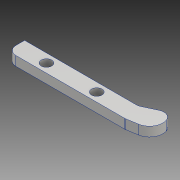
# Autodesk Inventor part: phalanx_1_tendon_support
Saved by Autodesk Inventor 2017 SP1 (Build 210196100, 196)
## iProperties
Created: 2017-07-31
Part Number: phalanx_1_tendon_support
Material: Aluminum 6061
Document SubType Name: Modeling
Designer: JT
Density: 2.7 g/cm^3
Appearance: Aluminum - Flat
Author: JT
Autodesk Inventor part; units mm, degrees
ref_plane "YZ Plane" through (0, 0, 0) normal (1, 0, 0) x (0, 1, 0)
ref_plane "XZ Plane" through (0, 0, 0) normal (0, 1, 0) x (-1, 0, 0)
ref_plane "XY Plane" through (0, 0, 0) normal (0, 0, 1) x (1, 0, 0)
sketch "Sketch1" plane through (0, 0, 0) normal (0, 0, 1) x (1, 0, 0)
  line L0 (0, 4) -> (0, 0) construction
  arc A0 (8.3449, 0.4035) -> (9.5, 6.1037) centre (8.2, 3.4) ccw
  line L1 (0, 0) -> (-21, 0)
  line L2 (-21, 0) -> (-21, 4)
  line L3 (0, 4) -> (0, 0)
  line L4 (-21, 4) -> (0, 4)
  line L5 (0, 4) -> (5, 4)
  line L6 (5, 4) -> (9.5, 6.1037)
  line L7 (0, 0) -> (6, 0)
  line L8 (6, 0) -> (8.6846, 0.4394)
  dimension "d0" = 8.2
  dimension "d1" = 3.4
  dimension "d3" = 6
  dimension "d47" = 21
  dimension "d57" = 4
  dimension "d66" = 5
  dimension "d67" = 9.5
  dimension "d68" = 6
  constraints: 18 end point, 4 horizontal, 3 point on circle, 1 centre point, 1 parallel, 1 perpendicular, 1 tangent
  measures "d0" distance from line of A0.centre L0
  measures "d1" vertical distance of L0.end A0.centre
  measures "d3" diameter of A0
  measures "d47" distance of L0.start L2.end
  measures "d57" distance between parallel lines of L1 L4
  measures "d66" distance of L0.start L5.end
  measures "d67" horizontal distance of L6.end L0.start
  measures "d68" distance of L0.end L7.end
extrude "Extrusion1" add sketch "Sketch1" along normal blind 2.15
sketch "Sketch6" plane through (0, 0, 0) normal (0, 0, -1) x (-1, 0, 0)
  arc A0 (-9.5, 6.1037) -> (-8.6846, 0.4394) centre (-8.2, 3.4) ccw projected
  point P0 (0, 0)
  point P1 (-3.5529, 0.4208)
  point P2 (-8.8532, 6.2809)
  point P3 (-10.6507, 0.558)
  constraints: 1 other
hole "Hole3" at (8.2, 3.4, 0) direction (0, 0, 1) diameter 1.5 depth 1.5 tip angle 118
sketch "Sketch7" plane through (0, 0, 0) normal (0, 0, -1) x (-1, 0, 0)
  circle A0 centre (-8.2, 3.4) radius 0.75 projected
  circle A1 centre (-8.2, 3.4) radius 1.1
  point P0 (0, 0)
  dimension "d44" = 2.2
  constraints: 1 centre point, 1 coincident
  measures "d44" diameter of A1
extrude "Extrusion4" add sketch "Sketch7" along normal blind 0.3
sketch "Sketch8" plane through (0, 0, 2.15) normal (0, 0, 1) x (1, 0, 0)
  arc A0 (8.6846, 0.4394) -> (9.5, 6.1037) centre (8.2, 3.4) ccw projected
  line L0 (-21, 4) -> (-21, 0) projected
  line L1 (-21, 4) -> (-21, 0) projected
  line L2 (-21, 2) -> (-1.49, 2) construction
  line L3 (5, 4) -> (-21, 4) projected
  line L4 (-21, 0) -> (6, 0) projected
  line L5 (6, 0) -> (8.6846, 0.4394) projected
  line L6 (9.5, 6.1037) -> (5, 4) projected
  point P0 (0, 0)
  point P1 (-14, 2)
  point P2 (-2.5, 2)
  dimension "d48" = 7
  dimension "d49" = 2.5
  constraints: 2 end point, 2 point on line, 1 horizontal, 1 midpoint
  measures "d48" distance from line of point (-14, 2) L0
  measures "d49" horizontal distance of point (-2.5, 2) point (0, 0)
hole "Hole4" at (-14, 2, 2.15) at (-2.5, 2, 2.15) direction (0, 0, -1) diameter 2.4 end through all
fillet "Fillet3" radius 2 1 edges at (9.5, 6.1037, 1.075)
fillet "Fillet5" radius 2 2 edges at (5, 4, 1.075) (6, 0, 1.075)
fillet "Fillet6" radius 2 1 edges at (-21, 0, 1.075)
body "Solid1"
